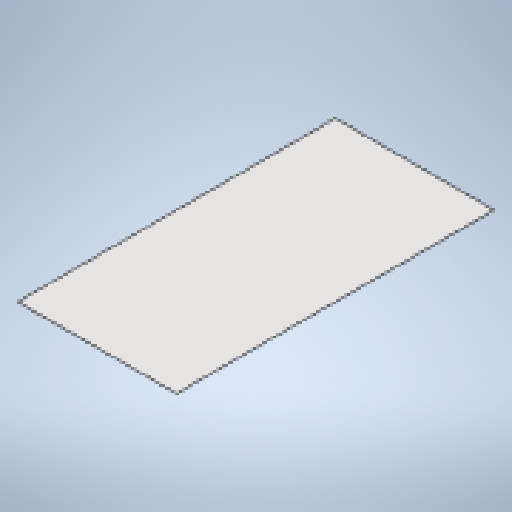
# Autodesk Inventor part: GhG frame1 floore sheet 1
Saved by Autodesk Inventor 2025.3 (Build 293356000, 356)
## iProperties
Created: 2025-10-28
Part Number: GhG frame1 floore sheet 1
Material: Stainless Steel
Document SubType Name: Sheet Metal
Designer: admin
Mass: 280.619 g
Surface Area: 364.406 cm^2
Volume: 35.0774 cm^3
Density: 8 g/cm^3
Sheet Metal Rule: AISI304 3mm Die 32
Sheet Metal Width: 0,000 mm
Sheet Metal Length: 0,000 mm
Sheet Metal Area: 0,000 mm^2
Appearance: Default
Author: admin
Autodesk Inventor part; units mm, degrees
ref_plane "YZ Plane" through (0, 0, 0) normal (1, 0, 0) x (0, 1, 0)
ref_plane "XZ Plane" through (0, 0, 0) normal (0, 1, 0) x (-1, 0, 0)
ref_plane "XY Plane" through (0, 0, 0) normal (0, 0, 1) x (1, 0, 0)
sketch "Sketch1" plane through (0, 0, 0) normal (0, 0, 1) x (1, 0, 0)
  line L0 (-625, -1050) -> (625, -1050)
  line L1 (625, -1050) -> (625, 1050)
  line L2 (625, 1050) -> (-625, 1050)
  line L3 (-625, 1050) -> (-625, -1050)
  line L4 (-625, -1050) -> (625, 1050) construction
  line L5 (625, -1050) -> (-625, 1050) construction
  line L6 (625, 1050) -> (590, 1050)
  line L7 (590, 1050) -> (590, 1015)
  line L8 (590, 1015) -> (625, 1015)
  line L9 (625, 1015) -> (625, 1050)
  point P0 (0, 0)
  dimension "d0" = 1250
  dimension "d1" = 2100
  dimension "d22" = 35
  dimension "d23" = 35
  measures "d0" distance of L2.end L1.end
  measures "d1" distance of L1.end L0.end
  measures "d22" distance of L8.end L7.end
  measures "d23" distance of L7.end L6.end
extrude "Plate1" add sketch "Sketch1" along normal blind 3
equation "\"d2\" = Thickness"
equation "\"BendReliefWidth\" = Thickness"
equation "\"BendReliefDepth\" = 0.5 * Thickness"
equation "\"CornerReliefSize\" = 4 * Thickness"
equation "\"MinimumRemnant\" = 2 * Thickness"
equation "\"TransitionRadius\" = BendRadius"
equation "\"JacobiRadiusSize\" = BendRadius"
equation "\"GapSize\" = Thickness"
equation "\"Thickness\" = 3"
equation "\"BendRadius\" = 5"
body "Solid1"
